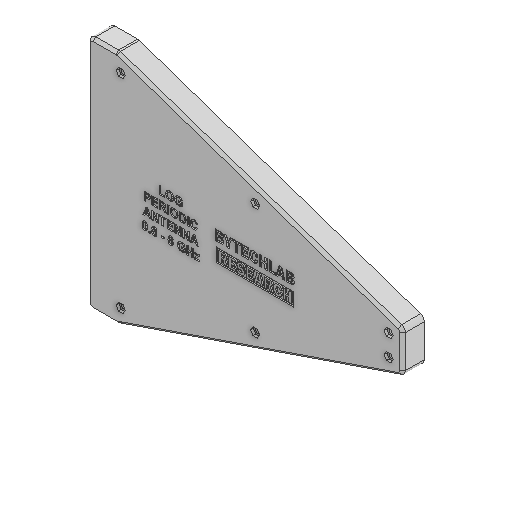
# Autodesk Inventor part: 3DP_PLA_Antenna_Case_Top
Saved by Autodesk Inventor 2026.1 (Build 301233000, 233)
## iProperties
Created: 2025-10-17
Part Number: 3DP_PLA_Antenna_Case_Top
Material: Generic
Document SubType Name: Modeling
Designer: User
Density: 1 g/cm^3
Appearance: Default
Author: User
Autodesk Inventor part; units mm, degrees
(part 1 of 2)
ref_plane "YZ Plane" through (0, 0, 0) normal (1, 0, 0) x (0, 1, 0)
ref_plane "XZ Plane" through (0, 0, 0) normal (0, 1, 0) x (-1, 0, 0)
ref_plane "XY Plane" through (0, 0, 0) normal (0, 0, 1) x (1, 0, 0)
sketch "Sketch1" plane through (0, 0, 0) normal (0, 0, 1) x (1, 0, 0)
  circle A0 centre (-98.0984, 74.6932) radius 1.75
  line L0 (-101.515, 79.4432) -> (103.485, 9.4432)
  circle A1 centre (1.4016, 40.6932) radius 1.75
  line L1 (103.485, 9.4432) -> (103.485, -10.5568)
  circle A2 centre (100.1516, -8.3068) radius 1.75
  line L2 (103.485, -10.5568) -> (-101.515, -80.5568)
  circle A3 centre (100.1516, 7.1932) radius 1.75
  circle A4 centre (1.4016, -41.8068) radius 1.75
  circle A5 centre (-98.0984, -75.8068) radius 1.75
  line L3 (-101.515, -80.5568) -> (-101.515, 79.4432)
  line L4 (106.5081, 11.581) -> (-101.5865, 82.6377)
  line L5 (-101.515, -83.7513) -> (106.5081, -12.719)
  line L6 (106.5081, -12.719) -> (106.5081, 11.581)
  line L7 (-101.5865, 82.6377) -> (-118.515, 82.6377)
  line L8 (-118.515, 82.6377) -> (-118.515, -83.7513)
  line L9 (-118.515, -83.7513) -> (-101.515, -83.7513)
  line L10 (-122.515, 86.6377) -> (-100.9224, 86.6377)
  line L11 (-100.9224, 86.6377) -> (110.5081, 14.4419)
  line L12 (110.5081, 14.4419) -> (110.5081, -15.5799)
  line L13 (110.5081, -15.5799) -> (-100.8509, -87.7513)
  line L14 (-100.8509, -87.7513) -> (-122.515, -87.7513)
  line L15 (-122.515, -87.7513) -> (-122.515, 86.6377)
  circle A6 centre (-98.0984, 74.6932) radius 6.5
  circle A7 centre (1.4016, 40.6932) radius 6.5
  circle A8 centre (100.1516, 7.1932) radius 6.5
  circle A9 centre (100.1516, -8.3068) radius 6.5
  circle A10 centre (1.4016, -41.8068) radius 6.5
  circle A11 centre (-98.0984, -75.8068) radius 6.5
  point P0 (-95.0293, -81.5366)
  point P1 (-97.022, -82.2171)
  point P2 (2.6291, -48.1898)
  point P3 (4.3345, -47.6075)
  point P4 (100.4087, -14.8017)
  point P5 (103.9207, -13.6025)
  point P6 (106.5081, -9.6655)
  point P7 (106.5081, -6.9481)
  point P8 (106.5081, 8.5519)
  point P9 (103.985, 12.4425)
  point P10 (100.3295, 13.6908)
  point P11 (106.5081, 5.8345)
  point P12 (4.4707, 46.423)
  point P13 (2.478, 47.1035)
  point P14 (-94.9118, 80.3585)
  point P15 (-97.1545, 81.1243)
  dimension "d0" = 205
  dimension "d1" = 160
  dimension "d2" = 20
  dimension "d3" = 71.147
  dimension "d4" = 3.4167
  dimension "d5" = 4.75
  dimension "d6" = 3.4167
  dimension "d7" = 4.75
  dimension "d8" = 38.75
  dimension "d9" = 72.25
  dimension "d10" = 102.9167
  dimension "d11" = 201.6667
  dimension "d12" = 201.6667
  dimension "d13" = 102.9167
  dimension "d14" = 38.75
  dimension "d15" = 72.25
  dimension "d16" = 3
  dimension "d18" = 17
  dimension "d19" = 4
  dimension "d24" = 13
  dimension "d25" = 13
  dimension "d26" = 13
  dimension "d27" = 13
  dimension "d28" = 13
  dimension "d29" = 13
  dimension "d33" = 3.5
  dimension "d34" = 3.5
  dimension "d35" = 3.5
  dimension "d36" = 3.5
  dimension "d37" = 3.5
  dimension "d38" = 3.5
  dimension "d64" = 17
  constraints: 32 end point, 12 centre point, 6 coincident, 4 perpendicular, 1 horizontal, 6 other
  measures "d0" distance between parallel lines of L1 L3
  measures "d1" distance of L2.end L0.start
  measures "d2" distance of L0.end L1.end
  measures "d3" angle of L3 L0
  measures "d4" distance from line of L3 A5.centre
  measures "d5" vertical distance of L2.end A5.centre
  measures "d6" distance from line of L3 A0.centre
  measures "d7" vertical distance of L0.start A0.centre
  measures "d8" vertical distance of A4.centre L2.end
  measures "d9" vertical distance of A2.centre L2.end
  measures "d10" distance from line of L3 A4.centre
  measures "d11" distance from line of L3 A2.centre
  measures "d12" distance from line of L3 A3.centre
  measures "d13" distance from line of L3 A1.centre
  measures "d14" vertical distance of A1.centre L0.start
  measures "d15" vertical distance of L0.start A3.centre
  measures "d16" distance between parallel lines of L0 L4
  measures "d18" distance between parallel lines of L3 L8
  measures "d19" distance between parallel lines of L7 L10
  measures "d24" diameter of A6
  measures "d25" diameter of A7
  measures "d26" diameter of A8
  measures "d27" diameter of A9
  measures "d28" diameter of A10
  measures "d29" diameter of A11
  measures "d33" diameter of A5
  measures "d34" diameter of A0
  measures "d35" diameter of A4
  measures "d36" diameter of A1
  measures "d37" diameter of A3
  measures "d38" diameter of A2
  measures "d64" distance of L8.end L5.start
extrude "Extrusion1" add sketch "Sketch1" along normal blind 3 contours L3 A6 L4 L0 | L0 A6 L3 | A6 L4 A7 L0 | L0 A7 A8 L1 A9 L2 A10 A11 L3 A6 | L3 A11 L5 L9 L8 L7 L4 A6 | A7 L4 L0 | L0 A7 | L4 A6 | A11 L2 L3 | L3 L2 A11 L5 | A7 L4 A8 L0 | A7 L4 | L5 A11 | A8 L4 L6 L1 L0 | L0 L1 A8 | L2 A10 L5 A11 | A8 L4 | A8 L6 A9 L1 | A10 L2 | L2 A10 L5 | L5 A10 | L4 L6 A8 | A9 L6 L5 L2 L1 | L1 L2 A9 | L6 A8 | L2 A9 L5 A10 | A9 L6 | L5 A9 | L6 L5 A9 | L10 L11 L12 L13 L14 L15
extrude "Extrusion2" add sketch "Sketch1" against normal blind 13 contours L4 A6 | A7 L4 | L5 A11 | A8 L4 | L5 A10 | L6 A8 | A9 L6 | L5 A9 | L10 L11 L12 L13 L14 L15
extrude "Extrusion3" add sketch "Sketch1" against normal blind 12.2 contours L3 A6 L4 L0 | L0 A6 L3 | A7 L4 L0 | L0 A7 | A11 L2 L3 | L3 L2 A11 L5 | A8 L4 L6 L1 L0 | L0 L1 A8 | A10 L2 | L2 A10 L5 | L4 L6 A8 | A9 L6 L5 L2 L1 | L1 L2 A9 | L6 L5 A9
fillet "Fillet1" radius 2 12 edges at (-95.0293, -81.5366, -6.1) (-97.022, -82.2171, -6.1) (4.3345, -47.6075, -6.1) (2.6291, -48.1898, -6.1) (100.4087, -14.8017, -6.1) (106.5081, -6.9481, -6.1) (106.5081, 5.8345, -6.1) (100.3295, 13.6908, -6.1) (2.478, 47.1035, -6.1) (4.4707, 46.423, -6.1) (-97.1545, 81.1243, -6.1) (-94.9118, 80.3585, -6.1)
sketch "Sketch2" plane through (-122.515, -87.7513, 3) normal (-1, 0, 0) x (0, 0, 1)
  line L0 (0, 0) -> (-16, 0) projected
  line L1 (0, 174.3889) -> (0, 0) projected
  line L2 (-16, 174.3889) -> (0, 174.3889) projected
  line L3 (-16, 0) -> (-16, 174.3889) projected
  circle A0 centre (-14.175, 87.1945) radius 3.15
  line L4 (-14.175, 84.0445) -> (-16, 84.0445)
  line L5 (-14.175, 90.3445) -> (-16, 90.3445)
  point P0 (-3, 87.7513)
  point P1 (-16, 84.627)
  point P2 (-16, 89.7619)
  dimension "d39" = 174.3889
  dimension "d40" = 87.1945
  dimension "d42" = 6.3
  dimension "d65" = 1.825
  constraints: 4 end point, 2 perpendicular, 2 point on circle, 2 point on line, 2 tangent, 1 centre point, 1 coincident
  measures "d39" distance of L0.end L2.start
  measures "d40" distance from line of L0 point (-14.175, 87.194)
  measures "d42" diameter of A0
  measures "d65" distance from line of L3 point (-14.175, 87.194)
extrude "Extrusion4" cut sketch "Sketch2" against normal blind 11.2 contours L3 A0 L4 | A0 L3 | L3 A0 | L5 A0 L3
fillet "Fillet2" radius 1.5 25 edges at (-2.0797, 47.5824, 0) (8.3695, 44.0144, 0) (-0.6988, 34.5419, 0) (52.7579, 29.9347, 0) (-46.2728, 63.7501, 0) (96.4821, 13.9532, 0) (94.9036, 3.3581, 0) (105.4955, 1.6337, 0) (-101.2403, 81.1736, 0) (-91.1224, 77.9902, 0) (-100.36, 68.5993, 0) (-110.0507, 82.6377, 0) (-118.515, -0.5568, 0) (-110.015, -83.7513, 0) (-46.2653, -64.8855, 0) (52.765, -31.0703, 0) (-100.3713, -69.7172, 0) (-91.1305, -79.128, 0) (-101.1979, -82.2945, 0) (8.3613, -45.1523, 0) (-2.0584, -48.7102, 0) (-0.6988, -35.6555, 0) (96.5027, -15.0813, 0) (94.8976, -4.4799, 0) (105.4955, -2.7473, 0)
sketch "Sketch4" plane through (0, 0, 3) normal (0, 0, 1) x (1, 0, 0)
  line L0 (-122.515, -87.7513) -> (-100.8509, -87.7513) projected
  line L1 (-100.8509, -87.7513) -> (110.5081, -15.5799) projected
  line L2 (110.5081, -15.5799) -> (110.5081, 14.4419) projected
  line L3 (110.5081, 14.4419) -> (-100.9224, 86.6377) projected
  line L4 (-100.9224, 86.6377) -> (-122.515, 86.6377) projected
  line L5 (-122.515, 86.6377) -> (-122.515, -87.7513) projected
  circle A0 centre (-98.0984, 74.6932) radius 1.75 projected
  circle A1 centre (1.4016, 40.6932) radius 1.75 projected
  circle A2 centre (-98.0984, -75.8068) radius 1.75 projected
  circle A3 centre (1.4016, -41.8068) radius 1.75 projected
  circle A4 centre (100.1516, -8.3068) radius 1.75 projected
  circle A5 centre (100.1516, 7.1932) radius 1.75 projected
  line L6 (-96.4385, 77.5682) -> (-94.7786, 74.6932)
  line L7 (-94.7786, 74.6932) -> (-96.4385, 71.8182)
  line L8 (-96.4385, 71.8182) -> (-99.7582, 71.8182)
  line L9 (-99.7582, 71.8182) -> (-101.4181, 74.6932)
  line L10 (-101.4181, 74.6932) -> (-99.7582, 77.5682)
  line L11 (-99.7582, 77.5682) -> (-96.4385, 77.5682)
  line L12 (3.0615, 43.5682) -> (4.7214, 40.6932)
  line L13 (4.7214, 40.6932) -> (3.0615, 37.8182)
  line L14 (3.0615, 37.8182) -> (-0.2582, 37.8182)
  line L15 (-0.2582, 37.8182) -> (-1.9181, 40.6932)
  line L16 (-1.9181, 40.6932) -> (-0.2582, 43.5682)
  line L17 (-0.2582, 43.5682) -> (3.0615, 43.5682)
  line L18 (101.8115, 10.0682) -> (103.4714, 7.1932)
  line L19 (103.4714, 7.1932) -> (101.8115, 4.3182)
  line L20 (101.8115, 4.3182) -> (98.4918, 4.3182)
  line L21 (98.4918, 4.3182) -> (96.8319, 7.1932)
  line L22 (96.8319, 7.1932) -> (98.4918, 10.0682)
  line L23 (98.4918, 10.0682) -> (101.8115, 10.0682)
  line L24 (101.8115, -5.4318) -> (103.4714, -8.3068)
  line L25 (103.4714, -8.3068) -> (101.8115, -11.1818)
  line L26 (101.8115, -11.1818) -> (98.4918, -11.1818)
  line L27 (98.4918, -11.1818) -> (96.8319, -8.3068)
  line L28 (96.8319, -8.3068) -> (98.4918, -5.4318)
  line L29 (98.4918, -5.4318) -> (101.8115, -5.4318)
  line L30 (3.0615, -38.9318) -> (4.7214, -41.8068)
  line L31 (4.7214, -41.8068) -> (3.0615, -44.6818)
  line L32 (3.0615, -44.6818) -> (-0.2582, -44.6818)
  line L33 (-0.2582, -44.6818) -> (-1.9181, -41.8068)
  line L34 (-1.9181, -41.8068) -> (-0.2582, -38.9318)
  line L35 (-0.2582, -38.9318) -> (3.0615, -38.9318)
  line L36 (-96.4385, -72.9318) -> (-94.7786, -75.8068)
  line L37 (-94.7786, -75.8068) -> (-96.4385, -78.6818)
  line L38 (-96.4385, -78.6818) -> (-99.7582, -78.6818)
  line L39 (-99.7582, -78.6818) -> (-101.4181, -75.8068)
  line L40 (-101.4181, -75.8068) -> (-99.7582, -72.9318)
  line L41 (-99.7582, -72.9318) -> (-96.4385, -72.9318)
  point P0 (0, 0)
  dimension "d66" = 5.75
  dimension "d67" = 5.75
  dimension "d68" = 5.75
  dimension "d69" = 5.75
  dimension "d70" = 5.75
  dimension "d71" = 5.75
  constraints: 72 end point, 6 coincident, 78 other
  measures "d66" distance between parallel lines of L38 L41
  measures "d67" distance between parallel lines of L35 L32
  measures "d68" distance between parallel lines of L29 L26
  measures "d69" distance between parallel lines of L23 L20
  measures "d70" distance between parallel lines of L14 L17
  measures "d71" distance between parallel lines of L8 L11
extrude "Extrusion5" cut sketch "Sketch4" against normal blind 2 contours L6 L7 L8 L9 L10 L11 | L12 L13 L14 L15 L16 L17 | L18 L19 L20 L21 L22 L23 | L24 L25 L26 L27 L28 L29 | L30 L31 L32 L33 L34 L35 | L36 L37 L38 L39 L40 L41
fillet "Fillet3" radius 4 10 edges at (-100.8509, -87.7513, -5) (110.5081, -15.5799, -5) (110.5081, 14.4419, -5) (-100.9224, 86.6377, -5) (-122.515, -87.7513, -5) (-122.515, 86.6377, -5) (-118.0757, 82.1983, -0.4393) (-118.515, 82.6377, -7.25) (-118.0757, -83.3119, -0.4393) (-118.515, -83.7513, -7.25)
chamfer "Chamfer1" distance 2 angle 45 12 edges at (3.7534, 50.8947, 3) (-100.9313, 86.5836, 3) (-110.0507, 86.6377, 3) (-121.3435, 85.4661, 3) (-122.515, -0.5568, 3) (-121.3435, -86.5797, 3) (-110.015, -87.7513, 3) (-100.8599, -87.6973, 3) (3.7891, -52.0205, 3) (109.7615, -15.046, 3) (110.5081, -0.569, 3) (109.7615, 13.908, 3)
sketch "Sketch6" plane through (0, 0, 3) normal (0, 0, 1) x (1, 0, 0)
  spline S0 degree 3 poles (-24.5157, 9.7786) (-23.8916, 9.7786) (-23.4226, 9.702) (-23.1087, 9.5487) knots 0 0 0 0 1 1 1 1
  line L0 (-24.5157, 9.7786) -> (-23.8916, 9.7786) construction
  line L1 (-23.8916, 9.7786) -> (-23.4226, 9.702) construction
  line L2 (-23.4226, 9.702) -> (-23.1087, 9.5487) construction
  spline S1 degree 3 poles (-23.1087, 9.5487) (-22.7948, 9.3954) (-22.5357, 9.1764) (-22.3313, 8.8917) knots 0 0 0 0 1 1 1 1
  line L3 (-23.1087, 9.5487) -> (-22.7948, 9.3954) construction
  line L4 (-22.7948, 9.3954) -> (-22.5357, 9.1764) construction
  line L5 (-22.5357, 9.1764) -> (-22.3313, 8.8917) construction
  spline S2 degree 3 poles (-22.3313, 8.8917) (-22.1269, 8.607) (-22.0247, 8.2602) (-22.0247, 7.8515) knots 0 0 0 0 1 1 1 1
  line L6 (-22.3313, 8.8917) -> (-22.1269, 8.607) construction
  line L7 (-22.1269, 8.607) -> (-22.0247, 8.2602) construction
  line L8 (-22.0247, 8.2602) -> (-22.0247, 7.8515) construction
  spline S3 degree 3 poles (-22.0247, 7.8515) (-22.0247, 7.0229) (-22.4736, 6.47) (-23.3715, 6.1926) knots 0 0 0 0 1 1 1 1
  line L9 (-22.0247, 7.8515) -> (-22.0247, 7.0229) construction
  line L10 (-22.0247, 7.0229) -> (-22.4736, 6.47) construction
  line L11 (-22.4736, 6.47) -> (-23.3715, 6.1926) construction
  spline S4 degree 3 poles (-23.3715, 6.1926) (-22.8532, 6.0758) (-22.4645, 5.844) (-22.2054, 5.4973) knots 0 0 0 0 1 1 1 1
  line L12 (-23.3715, 6.1926) -> (-22.8532, 6.0758) construction
  line L13 (-22.8532, 6.0758) -> (-22.4645, 5.844) construction
  line L14 (-22.4645, 5.844) -> (-22.2054, 5.4973) construction
  spline S5 degree 3 poles (-22.2054, 5.4973) (-21.9462, 5.1505) (-21.8166, 4.7728) (-21.8166, 4.364) knots 0 0 0 0 1 1 1 1
  line L15 (-22.2054, 5.4973) -> (-21.9462, 5.1505) construction
  line L16 (-21.9462, 5.1505) -> (-21.8166, 4.7728) construction
  line L17 (-21.8166, 4.7728) -> (-21.8166, 4.364) construction
  spline S6 degree 3 poles (-21.8166, 4.364) (-21.8166, 3.8055) (-22.0283, 3.3219) (-22.4517, 2.9131) knots 0 0 0 0 1 1 1 1
  line L18 (-21.8166, 4.364) -> (-21.8166, 3.8055) construction
  line L19 (-21.8166, 3.8055) -> (-22.0283, 3.3219) construction
  line L20 (-22.0283, 3.3219) -> (-22.4517, 2.9131) construction
  spline S7 degree 3 poles (-22.4517, 2.9131) (-22.8751, 2.508) (-23.5631, 2.3054) (-24.5157, 2.3054) knots 0 0 0 0 1 1 1 1
  line L21 (-22.4517, 2.9131) -> (-22.8751, 2.508) construction
  line L22 (-22.8751, 2.508) -> (-23.5631, 2.3054) construction
  line L23 (-23.5631, 2.3054) -> (-24.5157, 2.3054) construction
  line L24 (-27.9977, 9.7786) -> (-24.5157, 9.7786)
  line L25 (-24.5157, 2.3054) -> (-27.9977, 2.3054)
  line L26 (-27.9977, 2.3054) -> (-27.9977, 9.7786)
  spline S8 degree 3 poles (-24.9264, 6.8222) (-24.4409, 6.8222) (-24.1362, 6.9171) (-24.0121, 7.1069) knots 0 0 0 0 1 1 1 1
  line L27 (-24.9264, 6.8222) -> (-24.4409, 6.8222) construction
  line L28 (-24.4409, 6.8222) -> (-24.1362, 6.9171) construction
  line L29 (-24.1362, 6.9171) -> (-24.0121, 7.1069) construction
  spline S9 degree 3 poles (-24.0121, 7.1069) (-23.8843, 7.3003) (-23.8204, 7.4846) (-23.8204, 7.6598) knots 0 0 0 0 1 1 1 1
  line L30 (-24.0121, 7.1069) -> (-23.8843, 7.3003) construction
  line L31 (-23.8843, 7.3003) -> (-23.8204, 7.4846) construction
  line L32 (-23.8204, 7.4846) -> (-23.8204, 7.6598) construction
  spline S10 degree 3 poles (-23.8204, 7.6598) (-23.8204, 7.8496) (-23.8734, 8.012) (-23.9792, 8.1471) knots 0 0 0 0 1 1 1 1
  line L33 (-23.8204, 7.6598) -> (-23.8204, 7.8496) construction
  line L34 (-23.8204, 7.8496) -> (-23.8734, 8.012) construction
  line L35 (-23.8734, 8.012) -> (-23.9792, 8.1471) construction
  spline S11 degree 3 poles (-23.9792, 8.1471) (-24.0814, 8.2858) (-24.1946, 8.3716) (-24.3186, 8.4044) knots 0 0 0 0 1 1 1 1
  line L36 (-23.9792, 8.1471) -> (-24.0814, 8.2858) construction
  line L37 (-24.0814, 8.2858) -> (-24.1946, 8.3716) construction
  line L38 (-24.1946, 8.3716) -> (-24.3186, 8.4044) construction
  spline S12 degree 3 poles (-24.3186, 8.4044) (-24.4427, 8.4409) (-24.6873, 8.4592) (-25.0523, 8.4592) knots 0 0 0 0 1 1 1 1
  line L39 (-24.3186, 8.4044) -> (-24.4427, 8.4409) construction
  line L40 (-24.4427, 8.4409) -> (-24.6873, 8.4592) construction
  line L41 (-24.6873, 8.4592) -> (-25.0523, 8.4592) construction
  line L42 (-26.2513, 8.4592) -> (-26.2513, 6.8222)
  line L43 (-26.2513, 6.8222) -> (-24.9264, 6.8222)
  line L44 (-25.0523, 8.4592) -> (-26.2513, 8.4592)
  spline S13 degree 3 poles (-24.9045, 3.6906) (-24.4446, 3.6906) (-24.1197, 3.7709) (-23.9299, 3.9315) knots 0 0 0 0 1 1 1 1
  line L45 (-24.9045, 3.6906) -> (-24.4446, 3.6906) construction
  line L46 (-24.4446, 3.6906) -> (-24.1197, 3.7709) construction
  line L47 (-24.1197, 3.7709) -> (-23.9299, 3.9315) construction
  spline S14 degree 3 poles (-23.9299, 3.9315) (-23.7401, 4.0921) (-23.6452, 4.3165) (-23.6452, 4.6049) knots 0 0 0 0 1 1 1 1
  line L48 (-23.9299, 3.9315) -> (-23.7401, 4.0921) construction
  line L49 (-23.7401, 4.0921) -> (-23.6452, 4.3165) construction
  line L50 (-23.6452, 4.3165) -> (-23.6452, 4.6049) construction
  spline S15 degree 3 poles (-23.6452, 4.6049) (-23.6452, 4.8458) (-23.7365, 5.0538) (-23.919, 5.229) knots 0 0 0 0 1 1 1 1
  line L51 (-23.6452, 4.6049) -> (-23.6452, 4.8458) construction
  line L52 (-23.6452, 4.8458) -> (-23.7365, 5.0538) construction
  line L53 (-23.7365, 5.0538) -> (-23.919, 5.229) construction
  spline S16 degree 3 poles (-23.919, 5.229) (-24.1015, 5.4042) (-24.4044, 5.4918) (-24.8278, 5.4918) knots 0 0 0 0 1 1 1 1
  line L54 (-23.919, 5.229) -> (-24.1015, 5.4042) construction
  line L55 (-24.1015, 5.4042) -> (-24.4044, 5.4918) construction
  line L56 (-24.4044, 5.4918) -> (-24.8278, 5.4918) construction
  line L57 (-26.2513, 5.4918) -> (-26.2513, 3.6906)
  line L58 (-26.2513, 3.6906) -> (-24.9045, 3.6906)
  line L59 (-24.8278, 5.4918) -> (-26.2513, 5.4918)
  line L60 (-15.3946, 9.7786) -> (-17.7433, 5.4535)
  line L61 (-17.7433, 5.4535) -> (-17.7433, 2.3054)
  line L62 (-17.7433, 2.3054) -> (-19.4953, 2.3054)
  line L63 (-19.4953, 2.3054) -> (-19.4953, 5.4535)
  line L64 (-19.4953, 5.4535) -> (-21.844, 9.7786)
  line L65 (-21.844, 9.7786) -> (-19.8128, 9.7786)
  line L66 (-19.8128, 9.7786) -> (-18.3839, 6.9426)
  line L67 (-18.3839, 6.9426) -> (-16.9659, 9.7786)
  line L68 (-16.9659, 9.7786) -> (-15.3946, 9.7786)
  line L69 (-9.6844, 9.7786) -> (-9.6844, 8.3004)
  line L70 (-9.6844, 8.3004) -> (-11.5349, 8.3004)
  line L71 (-11.5349, 8.3004) -> (-11.5349, 2.3054)
  line L72 (-11.5349, 2.3054) -> (-13.3087, 2.3054)
  line L73 (-13.3087, 2.3054) -> (-13.3087, 8.3004)
  line L74 (-13.3087, 8.3004) -> (-15.1702, 8.3004)
  line L75 (-15.1702, 8.3004) -> (-15.1702, 9.7786)
  line L76 (-15.1702, 9.7786) -> (-9.6844, 9.7786)
  line L77 (-3.5963, 8.3551) -> (-7.1605, 8.3551)
  line L78 (-7.1605, 8.3551) -> (-7.1605, 6.8222)
  line L79 (-7.1605, 6.8222) -> (-4.3573, 6.8222)
  line L80 (-4.3573, 6.8222) -> (-4.3573, 5.4151)
  line L81 (-4.3573, 5.4151) -> (-7.1605, 5.4151)
  line L82 (-7.1605, 5.4151) -> (-7.1605, 3.7836)
  line L83 (-7.1605, 3.7836) -> (-3.5963, 3.7836)
  line L84 (-3.5963, 3.7836) -> (-3.5963, 2.3054)
  line L85 (-3.5963, 2.3054) -> (-8.9398, 2.3054)
  line L86 (-8.9398, 2.3054) -> (-8.9398, 9.7786)
  line L87 (-8.9398, 9.7786) -> (-3.5963, 9.7786)
  line L88 (-3.5963, 9.7786) -> (-3.5963, 8.3551)
  spline S17 degree 3 poles (1.6486, 6.8824) (1.623, 7.9372) (1.2124, 8.4646) (0.4167, 8.4646) knots 0 0 0 0 1 1 1 1
  line L89 (1.6486, 6.8824) -> (1.623, 7.9372) construction
  line L90 (1.623, 7.9372) -> (1.2124, 8.4646) construction
  line L91 (1.2124, 8.4646) -> (0.4167, 8.4646) construction
  spline S18 degree 3 poles (0.4167, 8.4646) (-0.4957, 8.4646) (-0.952, 7.6525) (-0.952, 6.0283) knots 0 0 0 0 1 1 1 1
  line L92 (0.4167, 8.4646) -> (-0.4957, 8.4646) construction
  line L93 (-0.4957, 8.4646) -> (-0.952, 7.6525) construction
  line L94 (-0.952, 7.6525) -> (-0.952, 6.0283) construction
  spline S19 degree 3 poles (-0.952, 6.0283) (-0.952, 5.0903) (-0.8279, 4.4534) (-0.5797, 4.1176) knots 0 0 0 0 1 1 1 1
  line L95 (-0.952, 6.0283) -> (-0.952, 5.0903) construction
  line L96 (-0.952, 5.0903) -> (-0.8279, 4.4534) construction
  line L97 (-0.8279, 4.4534) -> (-0.5797, 4.1176) construction
  spline S20 degree 3 poles (-0.5797, 4.1176) (-0.3315, 3.7855) (0.0153, 3.6194) (0.4605, 3.6194) knots 0 0 0 0 1 1 1 1
  line L98 (-0.5797, 4.1176) -> (-0.3315, 3.7855) construction
  line L99 (-0.3315, 3.7855) -> (0.0153, 3.6194) construction
  line L100 (0.0153, 3.6194) -> (0.4605, 3.6194) construction
  spline S21 degree 3 poles (0.4605, 3.6194) (1.1832, 3.6194) (1.6249, 4.0902) (1.7855, 5.0319) knots 0 0 0 0 1 1 1 1
  line L101 (0.4605, 3.6194) -> (1.1832, 3.6194) construction
  line L102 (1.1832, 3.6194) -> (1.6249, 4.0902) construction
  line L103 (1.6249, 4.0902) -> (1.7855, 5.0319) construction
  line L104 (3.4827, 6.9974) -> (1.6486, 6.8824)
  spline S22 degree 3 poles (3.4827, 4.9279) (3.3732, 4.0337) (3.0392, 3.3529) (2.4808, 2.8858) knots 0 0 0 0 1 1 1 1
  line L105 (3.4827, 4.9279) -> (3.3732, 4.0337) construction
  line L106 (3.3732, 4.0337) -> (3.0392, 3.3529) construction
  line L107 (3.0392, 3.3529) -> (2.4808, 2.8858) construction
  spline S23 degree 3 poles (2.4808, 2.8858) (1.926, 2.4222) (1.2453, 2.1905) (0.4386, 2.1905) knots 0 0 0 0 1 1 1 1
  line L108 (2.4808, 2.8858) -> (1.926, 2.4222) construction
  line L109 (1.926, 2.4222) -> (1.2453, 2.1905) construction
  line L110 (1.2453, 2.1905) -> (0.4386, 2.1905) construction
  spline S24 degree 3 poles (0.4386, 2.1905) (-0.5505, 2.1905) (-1.3553, 2.5317) (-1.9758, 3.2143) knots 0 0 0 0 1 1 1 1
  line L111 (0.4386, 2.1905) -> (-0.5505, 2.1905) construction
  line L112 (-0.5505, 2.1905) -> (-1.3553, 2.5317) construction
  line L113 (-1.3553, 2.5317) -> (-1.9758, 3.2143) construction
  spline S25 degree 3 poles (-1.9758, 3.2143) (-2.5926, 3.8968) (-2.901, 4.8403) (-2.901, 6.0448) knots 0 0 0 0 1 1 1 1
  line L114 (-1.9758, 3.2143) -> (-2.5926, 3.8968) construction
  line L115 (-2.5926, 3.8968) -> (-2.901, 4.8403) construction
  line L116 (-2.901, 4.8403) -> (-2.901, 6.0448) construction
  spline S26 degree 3 poles (-2.901, 6.0448) (-2.901, 7.1726) (-2.6017, 8.096) (-2.0031, 8.815) knots 0 0 0 0 1 1 1 1
  line L117 (-2.901, 6.0448) -> (-2.901, 7.1726) construction
  line L118 (-2.901, 7.1726) -> (-2.6017, 8.096) construction
  line L119 (-2.6017, 8.096) -> (-2.0031, 8.815) construction
  spline S27 degree 3 poles (-2.0031, 8.815) (-1.4046, 9.5341) (-0.587, 9.8936) (0.4496, 9.8936) knots 0 0 0 0 1 1 1 1
  line L120 (-2.0031, 8.815) -> (-1.4046, 9.5341) construction
  line L121 (-1.4046, 9.5341) -> (-0.587, 9.8936) construction
  line L122 (-0.587, 9.8936) -> (0.4496, 9.8936) construction
  spline S28 degree 3 poles (0.4496, 9.8936) (2.2453, 9.8936) (3.2564, 8.9282) (3.4827, 6.9974) knots 0 0 0 0 1 1 1 1
  line L123 (0.4496, 9.8936) -> (2.2453, 9.8936) construction
  line L124 (2.2453, 9.8936) -> (3.2564, 8.9282) construction
  line L125 (3.2564, 8.9282) -> (3.4827, 6.9974) construction
  line L126 (1.7855, 5.0319) -> (3.4827, 4.9279)
  line L127 (10.266, 9.7786) -> (10.266, 2.3054)
  line L128 (10.266, 2.3054) -> (8.5469, 2.3054)
  line L129 (8.5469, 2.3054) -> (8.5469, 5.3878)
  line L130 (8.5469, 5.3878) -> (6.2091, 5.3878)
  line L131 (6.2091, 5.3878) -> (6.2091, 2.3054)
  line L132 (6.2091, 2.3054) -> (4.49, 2.3054)
  line L133 (4.49, 2.3054) -> (4.49, 9.7786)
  line L134 (4.49, 9.7786) -> (6.2091, 9.7786)
  line L135 (6.2091, 9.7786) -> (6.2091, 6.866)
  line L136 (6.2091, 6.866) -> (8.5469, 6.866)
  line L137 (8.5469, 6.866) -> (8.5469, 9.7786)
  line L138 (8.5469, 9.7786) -> (10.266, 9.7786)
  line L139 (13.5345, 3.7836) -> (16.5073, 3.7836)
  line L140 (16.5073, 3.7836) -> (16.5073, 2.3054)
  line L141 (16.5073, 2.3054) -> (11.7606, 2.3054)
  line L142 (11.7606, 2.3054) -> (11.7606, 9.7786)
  line L143 (11.7606, 9.7786) -> (13.5345, 9.7786)
  line L144 (13.5345, 9.7786) -> (13.5345, 3.7836)
  line L145 (21.0788, 9.7786) -> (23.4166, 2.3054)
  line L146 (23.4166, 2.3054) -> (21.5333, 2.3054)
  line L147 (21.5333, 2.3054) -> (21.0788, 3.8439)
  line L148 (21.0788, 3.8439) -> (18.659, 3.8439)
  line L149 (18.659, 3.8439) -> (18.1881, 2.3054)
  line L150 (18.1881, 2.3054) -> (16.6552, 2.3054)
  line L151 (16.6552, 2.3054) -> (19.0477, 9.7786)
  line L152 (19.0477, 9.7786) -> (21.0788, 9.7786)
  line L153 (19.0805, 5.2235) -> (20.6682, 5.2235)
  line L154 (20.6682, 5.2235) -> (19.8744, 7.846)
  line L155 (19.8744, 7.846) -> (19.0805, 5.2235)
  spline S29 degree 3 poles (27.7034, 9.7786) (28.3276, 9.7786) (28.7966, 9.702) (29.1105, 9.5487) knots 0 0 0 0 1 1 1 1
  line L156 (27.7034, 9.7786) -> (28.3276, 9.7786) construction
  line L157 (28.3276, 9.7786) -> (28.7966, 9.702) construction
  line L158 (28.7966, 9.702) -> (29.1105, 9.5487) construction
  spline S30 degree 3 poles (29.1105, 9.5487) (29.4243, 9.3954) (29.6835, 9.1764) (29.8879, 8.8917) knots 0 0 0 0 1 1 1 1
  line L159 (29.1105, 9.5487) -> (29.4243, 9.3954) construction
  line L160 (29.4243, 9.3954) -> (29.6835, 9.1764) construction
  line L161 (29.6835, 9.1764) -> (29.8879, 8.8917) construction
  spline S31 degree 3 poles (29.8879, 8.8917) (30.0923, 8.607) (30.1945, 8.2602) (30.1945, 7.8515) knots 0 0 0 0 1 1 1 1
  line L162 (29.8879, 8.8917) -> (30.0923, 8.607) construction
  line L163 (30.0923, 8.607) -> (30.1945, 8.2602) construction
  line L164 (30.1945, 8.2602) -> (30.1945, 7.8515) construction
  spline S32 degree 3 poles (30.1945, 7.8515) (30.1945, 7.0229) (29.7455, 6.47) (28.8477, 6.1926) knots 0 0 0 0 1 1 1 1
  line L165 (30.1945, 7.8515) -> (30.1945, 7.0229) construction
  line L166 (30.1945, 7.0229) -> (29.7455, 6.47) construction
  line L167 (29.7455, 6.47) -> (28.8477, 6.1926) construction
  spline S33 degree 3 poles (28.8477, 6.1926) (29.3659, 6.0758) (29.7547, 5.844) (30.0138, 5.4973) knots 0 0 0 0 1 1 1 1
  line L168 (28.8477, 6.1926) -> (29.3659, 6.0758) construction
  line L169 (29.3659, 6.0758) -> (29.7547, 5.844) construction
  line L170 (29.7547, 5.844) -> (30.0138, 5.4973) construction
  spline S34 degree 3 poles (30.0138, 5.4973) (30.2729, 5.1505) (30.4025, 4.7728) (30.4025, 4.364) knots 0 0 0 0 1 1 1 1
  line L171 (30.0138, 5.4973) -> (30.2729, 5.1505) construction
  line L172 (30.2729, 5.1505) -> (30.4025, 4.7728) construction
  line L173 (30.4025, 4.7728) -> (30.4025, 4.364) construction
  spline S35 degree 3 poles (30.4025, 4.364) (30.4025, 3.8055) (30.1908, 3.3219) (29.7674, 2.9131) knots 0 0 0 0 1 1 1 1
  line L174 (30.4025, 4.364) -> (30.4025, 3.8055) construction
  line L175 (30.4025, 3.8055) -> (30.1908, 3.3219) construction
  line L176 (30.1908, 3.3219) -> (29.7674, 2.9131) construction
  spline S36 degree 3 poles (29.7674, 2.9131) (29.344, 2.508) (28.656, 2.3054) (27.7034, 2.3054) knots 0 0 0 0 1 1 1 1
  line L177 (29.7674, 2.9131) -> (29.344, 2.508) construction
  line L178 (29.344, 2.508) -> (28.656, 2.3054) construction
  line L179 (28.656, 2.3054) -> (27.7034, 2.3054) construction
  line L180 (24.2214, 9.7786) -> (27.7034, 9.7786)
  line L181 (27.7034, 2.3054) -> (24.2214, 2.3054)
  line L182 (24.2214, 2.3054) -> (24.2214, 9.7786)
  spline S37 degree 3 poles (27.2928, 6.8222) (27.7782, 6.8222) (28.083, 6.9171) (28.2071, 7.1069) knots 0 0 0 0 1 1 1 1
  line L183 (27.2928, 6.8222) -> (27.7782, 6.8222) construction
  line L184 (27.7782, 6.8222) -> (28.083, 6.9171) construction
  line L185 (28.083, 6.9171) -> (28.2071, 7.1069) construction
  spline S38 degree 3 poles (28.2071, 7.1069) (28.3349, 7.3003) (28.3987, 7.4846) (28.3987, 7.6598) knots 0 0 0 0 1 1 1 1
  line L186 (28.2071, 7.1069) -> (28.3349, 7.3003) construction
  line L187 (28.3349, 7.3003) -> (28.3987, 7.4846) construction
  line L188 (28.3987, 7.4846) -> (28.3987, 7.6598) construction
  spline S39 degree 3 poles (28.3987, 7.6598) (28.3987, 7.8496) (28.3458, 8.012) (28.24, 8.1471) knots 0 0 0 0 1 1 1 1
  line L189 (28.3987, 7.6598) -> (28.3987, 7.8496) construction
  line L190 (28.3987, 7.8496) -> (28.3458, 8.012) construction
  line L191 (28.3458, 8.012) -> (28.24, 8.1471) construction
  spline S40 degree 3 poles (28.24, 8.1471) (28.1378, 8.2858) (28.0246, 8.3716) (27.9005, 8.4044) knots 0 0 0 0 1 1 1 1
  line L192 (28.24, 8.1471) -> (28.1378, 8.2858) construction
  line L193 (28.1378, 8.2858) -> (28.0246, 8.3716) construction
  line L194 (28.0246, 8.3716) -> (27.9005, 8.4044) construction
  spline S41 degree 3 poles (27.9005, 8.4044) (27.7764, 8.4409) (27.5319, 8.4592) (27.1669, 8.4592) knots 0 0 0 0 1 1 1 1
  line L195 (27.9005, 8.4044) -> (27.7764, 8.4409) construction
  line L196 (27.7764, 8.4409) -> (27.5319, 8.4592) construction
  line L197 (27.5319, 8.4592) -> (27.1669, 8.4592) construction
  line L198 (25.9679, 8.4592) -> (25.9679, 6.8222)
  line L199 (25.9679, 6.8222) -> (27.2928, 6.8222)
  line L200 (27.1669, 8.4592) -> (25.9679, 8.4592)
  spline S42 degree 3 poles (27.3147, 3.6906) (27.7746, 3.6906) (28.0994, 3.7709) (28.2892, 3.9315) knots 0 0 0 0 1 1 1 1
  line L201 (27.3147, 3.6906) -> (27.7746, 3.6906) construction
  line L202 (27.7746, 3.6906) -> (28.0994, 3.7709) construction
  line L203 (28.0994, 3.7709) -> (28.2892, 3.9315) construction
  spline S43 degree 3 poles (28.2892, 3.9315) (28.479, 4.0921) (28.5739, 4.3165) (28.5739, 4.6049) knots 0 0 0 0 1 1 1 1
  line L204 (28.2892, 3.9315) -> (28.479, 4.0921) construction
  line L205 (28.479, 4.0921) -> (28.5739, 4.3165) construction
  line L206 (28.5739, 4.3165) -> (28.5739, 4.6049) construction
  spline S44 degree 3 poles (28.5739, 4.6049) (28.5739, 4.8458) (28.4827, 5.0538) (28.3002, 5.229) knots 0 0 0 0 1 1 1 1
  line L207 (28.5739, 4.6049) -> (28.5739, 4.8458) construction
  line L208 (28.5739, 4.8458) -> (28.4827, 5.0538) construction
  line L209 (28.4827, 5.0538) -> (28.3002, 5.229) construction
  spline S45 degree 3 poles (28.3002, 5.229) (28.1177, 5.4042) (27.8147, 5.4918) (27.3914, 5.4918) knots 0 0 0 0 1 1 1 1
  line L210 (28.3002, 5.229) -> (28.1177, 5.4042) construction
  line L211 (28.1177, 5.4042) -> (27.8147, 5.4918) construction
  line L212 (27.8147, 5.4918) -> (27.3914, 5.4918) construction
  line L213 (25.9679, 5.4918) -> (25.9679, 3.6906)
  line L214 (25.9679, 3.6906) -> (27.3147, 3.6906)
  line L215 (27.3914, 5.4918) -> (25.9679, 5.4918)
  line L216 (-27.4344, -1.5328) -> (29.8391, -1.5328)
  line L217 (29.8391, -1.5328) -> (29.8391, -11.3656)
  line L218 (29.8391, -11.3656) -> (-27.4344, -11.3656)
  line L219 (-27.4344, -11.3656) -> (-27.4344, -1.5328)
  spline S46 degree 3 poles (-22.2656, -2.7127) (-21.6597, -2.7127) (-21.1743, -2.7838) (-20.8093, -2.9262) knots 0 0 0 0 1 1 1 1
  line L220 (-22.2656, -2.7127) -> (-21.6597, -2.7127) construction
  line L221 (-21.6597, -2.7127) -> (-21.1743, -2.7838) construction
  line L222 (-21.1743, -2.7838) -> (-20.8093, -2.9262) construction
  spline S47 degree 3 poles (-20.8093, -2.9262) (-20.4406, -3.0649) (-20.1359, -3.3222) (-19.895, -3.6981) knots 0 0 0 0 1 1 1 1
  line L223 (-20.8093, -2.9262) -> (-20.4406, -3.0649) construction
  line L224 (-20.4406, -3.0649) -> (-20.1359, -3.3222) construction
  line L225 (-20.1359, -3.3222) -> (-19.895, -3.6981) construction
  spline S48 degree 3 poles (-19.895, -3.6981) (-19.6541, -4.0741) (-19.5336, -4.492) (-19.5336, -4.9519) knots 0 0 0 0 1 1 1 1
  line L226 (-19.895, -3.6981) -> (-19.6541, -4.0741) construction
  line L227 (-19.6541, -4.0741) -> (-19.5336, -4.492) construction
  line L228 (-19.5336, -4.492) -> (-19.5336, -4.9519) construction
  spline S49 degree 3 poles (-19.5336, -4.9519) (-19.5336, -5.8497) (-19.9661, -6.494) (-20.8312, -6.8845) knots 0 0 0 0 1 1 1 1
  line L229 (-19.5336, -4.9519) -> (-19.5336, -5.8497) construction
  line L230 (-19.5336, -5.8497) -> (-19.9661, -6.494) construction
  line L231 (-19.9661, -6.494) -> (-20.8312, -6.8845) construction
  line L232 (-23.7876, -7.2239) -> (-23.7876, -10.1858)
  line L233 (-23.7876, -10.1858) -> (-25.5505, -10.1858)
  line L234 (-25.5505, -10.1858) -> (-25.5505, -2.7127)
  line L235 (-25.5505, -2.7127) -> (-22.2656, -2.7127)
  line L236 (-20.8312, -6.8845) -> (-19.4515, -10.1858)
  line L237 (-19.4515, -10.1858) -> (-21.3841, -10.1858)
  line L238 (-21.3841, -10.1858) -> (-22.5338, -7.2239)
  line L239 (-22.5338, -7.2239) -> (-23.7876, -7.2239)
  spline S50 degree 3 poles (-22.7145, -5.9483) (-22.3641, -5.9483) (-22.1105, -5.9246) (-21.9535, -5.8771) knots 0 0 0 0 1 1 1 1
  line L240 (-22.7145, -5.9483) -> (-22.3641, -5.9483) construction
  line L241 (-22.3641, -5.9483) -> (-22.1105, -5.9246) construction
  line L242 (-22.1105, -5.9246) -> (-21.9535, -5.8771) construction
  spline S51 degree 3 poles (-21.9535, -5.8771) (-21.7929, -5.826) (-21.6506, -5.7165) (-21.5265, -5.5486) knots 0 0 0 0 1 1 1 1
  line L243 (-21.9535, -5.8771) -> (-21.7929, -5.826) construction
  line L244 (-21.7929, -5.826) -> (-21.6506, -5.7165) construction
  line L245 (-21.6506, -5.7165) -> (-21.5265, -5.5486) construction
  spline S52 degree 3 poles (-21.5265, -5.5486) (-21.4024, -5.3771) (-21.3403, -5.1818) (-21.3403, -4.9628) knots 0 0 0 0 1 1 1 1
  line L246 (-21.5265, -5.5486) -> (-21.4024, -5.3771) construction
  line L247 (-21.4024, -5.3771) -> (-21.3403, -5.1818) construction
  line L248 (-21.3403, -5.1818) -> (-21.3403, -4.9628) construction
  spline S53 degree 3 poles (-21.3403, -4.9628) (-21.3403, -4.7548) (-21.4024, -4.5686) (-21.5265, -4.4044) knots 0 0 0 0 1 1 1 1
  line L249 (-21.3403, -4.9628) -> (-21.3403, -4.7548) construction
  line L250 (-21.3403, -4.7548) -> (-21.4024, -4.5686) construction
  line L251 (-21.4024, -4.5686) -> (-21.5265, -4.4044) construction
  spline S54 degree 3 poles (-21.5265, -4.4044) (-21.6506, -4.2401) (-21.7856, -4.1398) (-21.9316, -4.1033) knots 0 0 0 0 1 1 1 1
  line L252 (-21.5265, -4.4044) -> (-21.6506, -4.2401) construction
  line L253 (-21.6506, -4.2401) -> (-21.7856, -4.1398) construction
  line L254 (-21.7856, -4.1398) -> (-21.9316, -4.1033) construction
  spline S55 degree 3 poles (-21.9316, -4.1033) (-22.0776, -4.0631) (-22.3513, -4.043) (-22.7528, -4.043) knots 0 0 0 0 1 1 1 1
  line L255 (-21.9316, -4.1033) -> (-22.0776, -4.0631) construction
  line L256 (-22.0776, -4.0631) -> (-22.3513, -4.043) construction
  line L257 (-22.3513, -4.043) -> (-22.7528, -4.043) construction
  line L258 (-23.7876, -4.043) -> (-23.7876, -5.9483)
  line L259 (-23.7876, -5.9483) -> (-22.7145, -5.9483)
  line L260 (-22.7528, -4.043) -> (-23.7876, -4.043)
  line L261 (-12.8434, -4.1361) -> (-16.4075, -4.1361)
  line L262 (-16.4075, -4.1361) -> (-16.4075, -5.6691)
  line L263 (-16.4075, -5.6691) -> (-13.6044, -5.6691)
  line L264 (-13.6044, -5.6691) -> (-13.6044, -7.0761)
  line L265 (-13.6044, -7.0761) -> (-16.4075, -7.0761)
  line L266 (-16.4075, -7.0761) -> (-16.4075, -8.7076)
  line L267 (-16.4075, -8.7076) -> (-12.8434, -8.7076)
  line L268 (-12.8434, -8.7076) -> (-12.8434, -10.1858)
  line L269 (-12.8434, -10.1858) -> (-18.1868, -10.1858)
  line L270 (-18.1868, -10.1858) -> (-18.1868, -2.7127)
  line L271 (-18.1868, -2.7127) -> (-12.8434, -2.7127)
  line L272 (-12.8434, -2.7127) -> (-12.8434, -4.1361)
  spline S56 degree 3 poles (-8.1186, -4.8533) (-8.3193, -4.262) (-8.7445, -3.9664) (-9.3942, -3.9664) knots 0 0 0 0 1 1 1 1
  line L273 (-8.1186, -4.8533) -> (-8.3193, -4.262) construction
  line L274 (-8.3193, -4.262) -> (-8.7445, -3.9664) construction
  line L275 (-8.7445, -3.9664) -> (-9.3942, -3.9664) construction
  spline S57 degree 3 poles (-9.3942, -3.9664) (-10.0877, -3.9664) (-10.4344, -4.1909) (-10.4344, -4.6398) knots 0 0 0 0 1 1 1 1
  line L276 (-9.3942, -3.9664) -> (-10.0877, -3.9664) construction
  line L277 (-10.0877, -3.9664) -> (-10.4344, -4.1909) construction
  line L278 (-10.4344, -4.1909) -> (-10.4344, -4.6398) construction
  spline S58 degree 3 poles (-10.4344, -4.6398) (-10.4344, -4.8187) (-10.3705, -4.9701) (-10.2428, -5.0942) knots 0 0 0 0 1 1 1 1
  line L279 (-10.4344, -4.6398) -> (-10.4344, -4.8187) construction
  line L280 (-10.4344, -4.8187) -> (-10.3705, -4.9701) construction
  line L281 (-10.3705, -4.9701) -> (-10.2428, -5.0942) construction
  spline S59 degree 3 poles (-10.2428, -5.0942) (-10.1114, -5.2183) (-9.8176, -5.326) (-9.3613, -5.4172) knots 0 0 0 0 1 1 1 1
  line L282 (-10.2428, -5.0942) -> (-10.1114, -5.2183) construction
  line L283 (-10.1114, -5.2183) -> (-9.8176, -5.326) construction
  line L284 (-9.8176, -5.326) -> (-9.3613, -5.4172) construction
  spline S60 degree 3 poles (-9.3613, -5.4172) (-8.5985, -5.5705) (-8.0401, -5.7257) (-7.686, -5.8826) knots 0 0 0 0 1 1 1 1
  line L285 (-9.3613, -5.4172) -> (-8.5985, -5.5705) construction
  line L286 (-8.5985, -5.5705) -> (-8.0401, -5.7257) construction
  line L287 (-8.0401, -5.7257) -> (-7.686, -5.8826) construction
  spline S61 degree 3 poles (-7.686, -5.8826) (-7.332, -6.0395) (-7.0345, -6.2932) (-6.7936, -6.6436) knots 0 0 0 0 1 1 1 1
  line L288 (-7.686, -5.8826) -> (-7.332, -6.0395) construction
  line L289 (-7.332, -6.0395) -> (-7.0345, -6.2932) construction
  line L290 (-7.0345, -6.2932) -> (-6.7936, -6.6436) construction
  spline S62 degree 3 poles (-6.7936, -6.6436) (-6.5491, -6.9903) (-6.4268, -7.3791) (-6.4268, -7.8097) knots 0 0 0 0 1 1 1 1
  line L291 (-6.7936, -6.6436) -> (-6.5491, -6.9903) construction
  line L292 (-6.5491, -6.9903) -> (-6.4268, -7.3791) construction
  line L293 (-6.4268, -7.3791) -> (-6.4268, -7.8097) construction
  spline S63 degree 3 poles (-6.4268, -7.8097) (-6.4268, -8.485) (-6.6878, -9.069) (-7.2097, -9.5617) knots 0 0 0 0 1 1 1 1
  line L294 (-6.4268, -7.8097) -> (-6.4268, -8.485) construction
  line L295 (-6.4268, -8.485) -> (-6.6878, -9.069) construction
  line L296 (-6.6878, -9.069) -> (-7.2097, -9.5617) construction
  spline S64 degree 3 poles (-7.2097, -9.5617) (-7.728, -10.0544) (-8.4981, -10.3008) (-9.5201, -10.3008) knots 0 0 0 0 1 1 1 1
  line L297 (-7.2097, -9.5617) -> (-7.728, -10.0544) construction
  line L298 (-7.728, -10.0544) -> (-8.4981, -10.3008) construction
  line L299 (-8.4981, -10.3008) -> (-9.5201, -10.3008) construction
  spline S65 degree 3 poles (-9.5201, -10.3008) (-10.2866, -10.3008) (-10.9399, -10.1274) (-11.4801, -9.7807) knots 0 0 0 0 1 1 1 1
  line L300 (-9.5201, -10.3008) -> (-10.2866, -10.3008) construction
  line L301 (-10.2866, -10.3008) -> (-10.9399, -10.1274) construction
  line L302 (-10.9399, -10.1274) -> (-11.4801, -9.7807) construction
  spline S66 degree 3 poles (-11.4801, -9.7807) (-12.0167, -9.4303) (-12.3707, -8.912) (-12.5422, -8.2258) knots 0 0 0 0 1 1 1 1
  line L303 (-11.4801, -9.7807) -> (-12.0167, -9.4303) construction
  line L304 (-12.0167, -9.4303) -> (-12.3707, -8.912) construction
  line L305 (-12.3707, -8.912) -> (-12.5422, -8.2258) construction
  line L306 (-6.6294, -4.3551) -> (-8.1186, -4.8533)
  spline S67 degree 3 poles (-10.9217, -7.859) (-10.7392, -8.5562) (-10.2318, -8.9047) (-9.3997, -8.9047) knots 0 0 0 0 1 1 1 1
  line L307 (-10.9217, -7.859) -> (-10.7392, -8.5562) construction
  line L308 (-10.7392, -8.5562) -> (-10.2318, -8.9047) construction
  line L309 (-10.2318, -8.9047) -> (-9.3997, -8.9047) construction
  spline S68 degree 3 poles (-9.3997, -8.9047) (-8.9982, -8.9047) (-8.6989, -8.8281) (-8.5018, -8.6748) knots 0 0 0 0 1 1 1 1
  line L310 (-9.3997, -8.9047) -> (-8.9982, -8.9047) construction
  line L311 (-8.9982, -8.9047) -> (-8.6989, -8.8281) construction
  line L312 (-8.6989, -8.8281) -> (-8.5018, -8.6748) construction
  spline S69 degree 3 poles (-8.5018, -8.6748) (-8.3047, -8.5178) (-8.2062, -8.3317) (-8.2062, -8.1163) knots 0 0 0 0 1 1 1 1
  line L313 (-8.5018, -8.6748) -> (-8.3047, -8.5178) construction
  line L314 (-8.3047, -8.5178) -> (-8.2062, -8.3317) construction
  line L315 (-8.2062, -8.3317) -> (-8.2062, -8.1163) construction
  spline S70 degree 3 poles (-8.2062, -8.1163) (-8.2062, -7.8973) (-8.2956, -7.7276) (-8.4744, -7.6072) knots 0 0 0 0 1 1 1 1
  line L316 (-8.2062, -8.1163) -> (-8.2062, -7.8973) construction
  line L317 (-8.2062, -7.8973) -> (-8.2956, -7.7276) construction
  line L318 (-8.2956, -7.7276) -> (-8.4744, -7.6072) construction
  spline S71 degree 3 poles (-8.4744, -7.6072) (-8.6533, -7.4867) (-8.9982, -7.3736) (-9.5092, -7.2677) knots 0 0 0 0 1 1 1 1
  line L319 (-8.4744, -7.6072) -> (-8.6533, -7.4867) construction
  line L320 (-8.6533, -7.4867) -> (-8.9982, -7.3736) construction
  line L321 (-8.9982, -7.3736) -> (-9.5092, -7.2677) construction
  spline S72 degree 3 poles (-9.5092, -7.2677) (-10.4618, -7.0706) (-11.1407, -6.8024) (-11.5458, -6.4629) knots 0 0 0 0 1 1 1 1
  line L322 (-9.5092, -7.2677) -> (-10.4618, -7.0706) construction
  line L323 (-10.4618, -7.0706) -> (-11.1407, -6.8024) construction
  line L324 (-11.1407, -6.8024) -> (-11.5458, -6.4629) construction
  spline S73 degree 3 poles (-11.5458, -6.4629) (-11.951, -6.1198) (-12.1535, -5.6198) (-12.1535, -4.9628) knots 0 0 0 0 1 1 1 1
  line L325 (-11.5458, -6.4629) -> (-11.951, -6.1198) construction
  line L326 (-11.951, -6.1198) -> (-12.1535, -5.6198) construction
  line L327 (-12.1535, -5.6198) -> (-12.1535, -4.9628) construction
  spline S74 degree 3 poles (-12.1535, -4.9628) (-12.1535, -4.2985) (-11.9126, -3.7383) (-11.4308, -3.282) knots 0 0 0 0 1 1 1 1
  line L328 (-12.1535, -4.9628) -> (-12.1535, -4.2985) construction
  line L329 (-12.1535, -4.2985) -> (-11.9126, -3.7383) construction
  line L330 (-11.9126, -3.7383) -> (-11.4308, -3.282) construction
  spline S75 degree 3 poles (-11.4308, -3.282) (-10.9454, -2.8258) (-10.2884, -2.5977) (-9.4599, -2.5977) knots 0 0 0 0 1 1 1 1
  line L331 (-11.4308, -3.282) -> (-10.9454, -2.8258) construction
  line L332 (-10.9454, -2.8258) -> (-10.2884, -2.5977) construction
  line L333 (-10.2884, -2.5977) -> (-9.4599, -2.5977) construction
  spline S76 degree 3 poles (-9.4599, -2.5977) (-7.9926, -2.5977) (-7.0491, -3.1835) (-6.6294, -4.3551) knots 0 0 0 0 1 1 1 1
  line L334 (-9.4599, -2.5977) -> (-7.9926, -2.5977) construction
  line L335 (-7.9926, -2.5977) -> (-7.0491, -3.1835) construction
  line L336 (-7.0491, -3.1835) -> (-6.6294, -4.3551) construction
  line L337 (-12.5422, -8.2258) -> (-10.9217, -7.859)
  line L338 (0.0554, -4.1361) -> (-3.5087, -4.1361)
  line L339 (-3.5087, -4.1361) -> (-3.5087, -5.6691)
  line L340 (-3.5087, -5.6691) -> (-0.7056, -5.6691)
  line L341 (-0.7056, -5.6691) -> (-0.7056, -7.0761)
  line L342 (-0.7056, -7.0761) -> (-3.5087, -7.0761)
  line L343 (-3.5087, -7.0761) -> (-3.5087, -8.7076)
  line L344 (-3.5087, -8.7076) -> (0.0554, -8.7076)
  line L345 (0.0554, -8.7076) -> (0.0554, -10.1858)
  line L346 (0.0554, -10.1858) -> (-5.2881, -10.1858)
  line L347 (-5.2881, -10.1858) -> (-5.2881, -2.7127)
  line L348 (-5.2881, -2.7127) -> (0.0554, -2.7127)
  line L349 (0.0554, -2.7127) -> (0.0554, -4.1361)
  line L350 (4.7802, -2.7127) -> (7.118, -10.1858)
  line L351 (7.118, -10.1858) -> (5.2346, -10.1858)
  line L352 (5.2346, -10.1858) -> (4.7802, -8.6474)
  line L353 (4.7802, -8.6474) -> (2.3603, -8.6474)
  line L354 (2.3603, -8.6474) -> (1.8895, -10.1858)
  line L355 (1.8895, -10.1858) -> (0.3565, -10.1858)
  line L356 (0.3565, -10.1858) -> (2.749, -2.7127)
  line L357 (2.749, -2.7127) -> (4.7802, -2.7127)
  line L358 (2.7819, -7.2677) -> (4.3696, -7.2677)
  line L359 (4.3696, -7.2677) -> (3.5757, -4.6453)
  line L360 (3.5757, -4.6453) -> (2.7819, -7.2677)
  spline S77 degree 3 poles (11.2077, -2.7127) (11.8136, -2.7127) (12.299, -2.7838) (12.664, -2.9262) knots 0 0 0 0 1 1 1 1
  line L361 (11.2077, -2.7127) -> (11.8136, -2.7127) construction
  line L362 (11.8136, -2.7127) -> (12.299, -2.7838) construction
  line L363 (12.299, -2.7838) -> (12.664, -2.9262) construction
  spline S78 degree 3 poles (12.664, -2.9262) (13.0326, -3.0649) (13.3374, -3.3222) (13.5783, -3.6981) knots 0 0 0 0 1 1 1 1
  line L364 (12.664, -2.9262) -> (13.0326, -3.0649) construction
  line L365 (13.0326, -3.0649) -> (13.3374, -3.3222) construction
  line L366 (13.3374, -3.3222) -> (13.5783, -3.6981) construction
  spline S79 degree 3 poles (13.5783, -3.6981) (13.8192, -4.0741) (13.9396, -4.492) (13.9396, -4.9519) knots 0 0 0 0 1 1 1 1
  line L367 (13.5783, -3.6981) -> (13.8192, -4.0741) construction
  line L368 (13.8192, -4.0741) -> (13.9396, -4.492) construction
  line L369 (13.9396, -4.492) -> (13.9396, -4.9519) construction
  spline S80 degree 3 poles (13.9396, -4.9519) (13.9396, -5.8497) (13.5071, -6.494) (12.6421, -6.8845) knots 0 0 0 0 1 1 1 1
  line L370 (13.9396, -4.9519) -> (13.9396, -5.8497) construction
  line L371 (13.9396, -5.8497) -> (13.5071, -6.494) construction
  line L372 (13.5071, -6.494) -> (12.6421, -6.8845) construction
  line L373 (9.6857, -7.2239) -> (9.6857, -10.1858)
  line L374 (9.6857, -10.1858) -> (7.9228, -10.1858)
  line L375 (7.9228, -10.1858) -> (7.9228, -2.7127)
  line L376 (7.9228, -2.7127) -> (11.2077, -2.7127)
  line L377 (12.6421, -6.8845) -> (14.0218, -10.1858)
  line L378 (14.0218, -10.1858) -> (12.0891, -10.1858)
  line L379 (12.0891, -10.1858) -> (10.9394, -7.2239)
  line L380 (10.9394, -7.2239) -> (9.6857, -7.2239)
  spline S81 degree 3 poles (10.7587, -5.9483) (11.1091, -5.9483) (11.3628, -5.9246) (11.5197, -5.8771) knots 0 0 0 0 1 1 1 1
  line L381 (10.7587, -5.9483) -> (11.1091, -5.9483) construction
  line L382 (11.1091, -5.9483) -> (11.3628, -5.9246) construction
  line L383 (11.3628, -5.9246) -> (11.5197, -5.8771) construction
  spline S82 degree 3 poles (11.5197, -5.8771) (11.6803, -5.826) (11.8227, -5.7165) (11.9468, -5.5486) knots 0 0 0 0 1 1 1 1
  line L384 (11.5197, -5.8771) -> (11.6803, -5.826) construction
  line L385 (11.6803, -5.826) -> (11.8227, -5.7165) construction
  line L386 (11.8227, -5.7165) -> (11.9468, -5.5486) construction
  spline S83 degree 3 poles (11.9468, -5.5486) (12.0709, -5.3771) (12.1329, -5.1818) (12.1329, -4.9628) knots 0 0 0 0 1 1 1 1
  line L387 (11.9468, -5.5486) -> (12.0709, -5.3771) construction
  line L388 (12.0709, -5.3771) -> (12.1329, -5.1818) construction
  line L389 (12.1329, -5.1818) -> (12.1329, -4.9628) construction
  spline S84 degree 3 poles (12.1329, -4.9628) (12.1329, -4.7548) (12.0709, -4.5686) (11.9468, -4.4044) knots 0 0 0 0 1 1 1 1
  line L390 (12.1329, -4.9628) -> (12.1329, -4.7548) construction
  line L391 (12.1329, -4.7548) -> (12.0709, -4.5686) construction
  line L392 (12.0709, -4.5686) -> (11.9468, -4.4044) construction
  spline S85 degree 3 poles (11.9468, -4.4044) (11.8227, -4.2401) (11.6876, -4.1398) (11.5416, -4.1033) knots 0 0 0 0 1 1 1 1
  line L393 (11.9468, -4.4044) -> (11.8227, -4.2401) construction
  line L394 (11.8227, -4.2401) -> (11.6876, -4.1398) construction
  line L395 (11.6876, -4.1398) -> (11.5416, -4.1033) construction
  spline S86 degree 3 poles (11.5416, -4.1033) (11.3957, -4.0631) (11.1219, -4.043) (10.7204, -4.043) knots 0 0 0 0 1 1 1 1
  line L396 (11.5416, -4.1033) -> (11.3957, -4.0631) construction
  line L397 (11.3957, -4.0631) -> (11.1219, -4.043) construction
  line L398 (11.1219, -4.043) -> (10.7204, -4.043) construction
  line L399 (9.6857, -4.043) -> (9.6857, -5.9483)
  line L400 (9.6857, -5.9483) -> (10.7587, -5.9483)
  line L401 (10.7204, -4.043) -> (9.6857, -4.043)
  spline S87 degree 3 poles (19.3378, -5.6089) (19.3123, -4.554) (18.9017, -4.0266) (18.106, -4.0266) knots 0 0 0 0 1 1 1 1
  line L402 (19.3378, -5.6089) -> (19.3123, -4.554) construction
  line L403 (19.3123, -4.554) -> (18.9017, -4.0266) construction
  line L404 (18.9017, -4.0266) -> (18.106, -4.0266) construction
  spline S88 degree 3 poles (18.106, -4.0266) (17.1935, -4.0266) (16.7373, -4.8387) (16.7373, -6.4629) knots 0 0 0 0 1 1 1 1
  line L405 (18.106, -4.0266) -> (17.1935, -4.0266) construction
  line L406 (17.1935, -4.0266) -> (16.7373, -4.8387) construction
  line L407 (16.7373, -4.8387) -> (16.7373, -6.4629) construction
  spline S89 degree 3 poles (16.7373, -6.4629) (16.7373, -7.401) (16.8614, -8.0379) (17.1096, -8.3737) knots 0 0 0 0 1 1 1 1
  line L408 (16.7373, -6.4629) -> (16.7373, -7.401) construction
  line L409 (16.7373, -7.401) -> (16.8614, -8.0379) construction
  line L410 (16.8614, -8.0379) -> (17.1096, -8.3737) construction
  spline S90 degree 3 poles (17.1096, -8.3737) (17.3578, -8.7058) (17.7045, -8.8719) (18.1498, -8.8719) knots 0 0 0 0 1 1 1 1
  line L411 (17.1096, -8.3737) -> (17.3578, -8.7058) construction
  line L412 (17.3578, -8.7058) -> (17.7045, -8.8719) construction
  line L413 (17.7045, -8.8719) -> (18.1498, -8.8719) construction
  spline S91 degree 3 poles (18.1498, -8.8719) (18.8725, -8.8719) (19.3141, -8.401) (19.4747, -7.4594) knots 0 0 0 0 1 1 1 1
  line L414 (18.1498, -8.8719) -> (18.8725, -8.8719) construction
  line L415 (18.8725, -8.8719) -> (19.3141, -8.401) construction
  line L416 (19.3141, -8.401) -> (19.4747, -7.4594) construction
  line L417 (21.1719, -5.4939) -> (19.3378, -5.6089)
  spline S92 degree 3 poles (21.1719, -7.5634) (21.0624, -8.4576) (20.7285, -9.1383) (20.17, -9.6055) knots 0 0 0 0 1 1 1 1
  line L418 (21.1719, -7.5634) -> (21.0624, -8.4576) construction
  line L419 (21.0624, -8.4576) -> (20.7285, -9.1383) construction
  line L420 (20.7285, -9.1383) -> (20.17, -9.6055) construction
  spline S93 degree 3 poles (20.17, -9.6055) (19.6152, -10.069) (18.9345, -10.3008) (18.1279, -10.3008) knots 0 0 0 0 1 1 1 1
  line L421 (20.17, -9.6055) -> (19.6152, -10.069) construction
  line L422 (19.6152, -10.069) -> (18.9345, -10.3008) construction
  line L423 (18.9345, -10.3008) -> (18.1279, -10.3008) construction
  spline S94 degree 3 poles (18.1279, -10.3008) (17.1388, -10.3008) (16.334, -9.9595) (15.7135, -9.277) knots 0 0 0 0 1 1 1 1
  line L424 (18.1279, -10.3008) -> (17.1388, -10.3008) construction
  line L425 (17.1388, -10.3008) -> (16.334, -9.9595) construction
  line L426 (16.334, -9.9595) -> (15.7135, -9.277) construction
  spline S95 degree 3 poles (15.7135, -9.277) (15.0967, -8.5945) (14.7882, -7.651) (14.7882, -6.4465) knots 0 0 0 0 1 1 1 1
  line L427 (15.7135, -9.277) -> (15.0967, -8.5945) construction
  line L428 (15.0967, -8.5945) -> (14.7882, -7.651) construction
  line L429 (14.7882, -7.651) -> (14.7882, -6.4465) construction